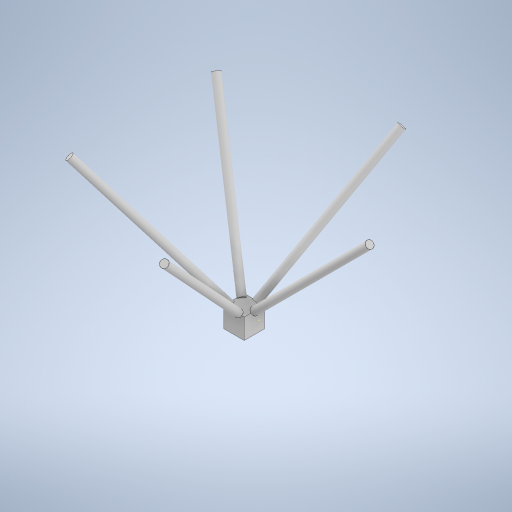
# Autodesk Inventor part: Part1
Saved by Autodesk Inventor 2024 (Build 280153020, 153B)
## iProperties
Created: 2023-11-21
Part Number: Part1
Material: Generic
Document SubType Name: Modeling
Designer: 5802269
Density: 1 g/cm^3
Appearance: Default
Author: 5802269
Autodesk Inventor part; units mm, degrees
ref_plane "YZ Plane" through (0, 0, 0) normal (1, 0, 0) x (0, 1, 0)
ref_plane "XZ Plane" through (0, 0, 0) normal (0, 1, 0) x (-1, 0, 0)
ref_plane "XY Plane" through (0, 0, 0) normal (0, 0, 1) x (1, 0, 0)
sketch "Sketch3" plane through (0, 0, 0) normal (0, 1, 0) x (-1, 0, 0)
  line L0 (-12.061, 12.1008) -> (12.939, 12.1008)
  line L1 (12.939, 12.1008) -> (12.939, -12.8992)
  line L2 (12.939, -12.8992) -> (-12.061, -12.8992)
  line L3 (-12.061, -12.8992) -> (-12.061, 12.1008)
  line L4 (-12.061, 12.1008) -> (12.939, -12.8992) construction
  line L5 (12.939, 12.1008) -> (-12.061, -12.8992) construction
  point P0 (0, 0)
  point P1 (0.439, -0.3992)
  dimension "d4" = 25
  dimension "d5" = 25
  constraints: 12 end point, 2 midpoint, 2 parallel, 1 horizontal, 1 perpendicular
  measures "d4" distance of L1.end L2.end
  measures "d5" distance of L0.end L1.end
extrude "Extrusion2" add sketch "Sketch3" along normal blind 25
ref_plane "Work Plane1" through (12.061, 25, 12.1008) normal (0.7071068, 0.7071068, 0) x (0, 0, -1)
sketch "Sketch4" plane through (12.061, 25, 12.1008) normal (0.7071068, 0.7071068, 0) x (0, 0, -1)
  line L0 (0, 0) -> (25, 0) projected
  circle A0 centre (12.5, 0) radius 4.5
  point P0 (12.1008, -9.1492)
  dimension "d9" = 9
  constraints: 1 centre point, 1 midpoint
  measures "d9" diameter of A0
sketch "Sketch5" plane through (12.061, 25, 12.1008) normal (0.7071068, 0.7071068, 0) x (0, 0, -1)
  point P0 (12.1008, -9.1492)
extrude "Extrusion3" add sketch "Sketch4" along normal blind 200
pattern_circular "Circular Pattern1" count 5 over 360 about axis through (0, -10, 0) along (0, 1, 0) of "Extrusion3"
body "Solid2"
